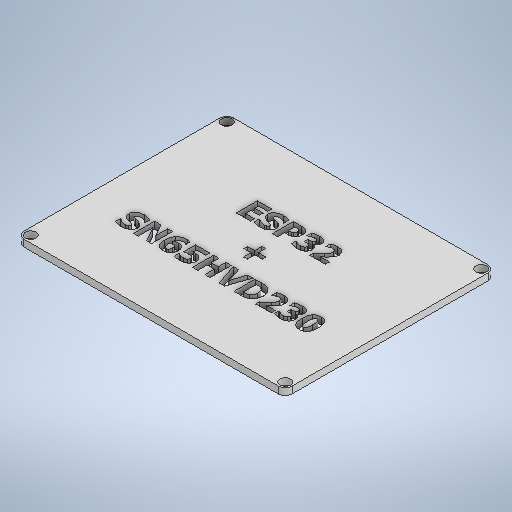
# Autodesk Inventor part: esp_can_case_lid
Saved by Autodesk Inventor 2025 (Build 290162000, 162)
## iProperties
Created: 2025-01-20
Part Number: esp_can_case_lid
Material: Generic
Document SubType Name: Modeling
Designer: danielrachi
Density: 1 g/cm^3
Appearance: Default
Author: danielrachi
Autodesk Inventor part; units mm, degrees
ref_plane "YZ Plane" through (0, 0, 0) normal (1, 0, 0) x (0, 1, 0)
ref_plane "XZ Plane" through (0, 0, 0) normal (0, 1, 0) x (-1, 0, 0)
ref_plane "XY Plane" through (0, 0, 0) normal (0, 0, 1) x (1, 0, 0)
sketch "Sketch1" plane through (0, 0, 0) normal (0, 1, 0) x (-1, 0, 0)
  line L0 (-39, 30.5) -> (39, 30.5)
  line L1 (39, 30.5) -> (39, -30.5)
  line L2 (39, -30.5) -> (-39, -30.5)
  line L3 (-39, -30.5) -> (-39, 30.5)
  line L4 (-39, 30.5) -> (39, -30.5) construction
  line L5 (39, 30.5) -> (-39, -30.5) construction
  point P0 (0, 0)
  dimension "d0" = 78
  dimension "d1" = 61
  constraints: 12 end point, 2 midpoint, 2 parallel, 1 horizontal, 1 perpendicular
  measures "d0" distance of L1.end L2.end
  measures "d1" distance of L0.end L1.end
extrude "Extrusion1" add sketch "Sketch1" along normal blind 2
sketch "Sketch2" plane through (0, 2, 0) normal (0, 1, 0) x (1, 0, 0)
  circle A0 centre (37, -28.5) radius 1.55
  line L0 (-39, -30.5) -> (39, -30.5) projected
  line L1 (39, -30.5) -> (39, 30.5) projected
  line L2 (-39, 30.5) -> (-39, -30.5) projected
  line L3 (-39, 0) -> (39, 0)
  line L4 (39, 30.5) -> (-39, 30.5) projected
  line L5 (0, 30.5) -> (0, -30.5)
  circle A1 centre (-37, -28.5) radius 1.55
  circle A2 centre (37, 28.5) radius 1.55
  circle A3 centre (-37, 28.5) radius 1.55
  line L6 (-39, 30.5) -> (39, 30.5) construction
  line L7 (39, 30.5) -> (39, -30.5) construction
  line L8 (39, -30.5) -> (-39, -30.5) construction
  line L9 (-39, -30.5) -> (-39, 30.5) construction
  line L10 (-12.7042, 6.9935) -> (-12.7042, 13.0935)
  line L11 (-12.7042, 13.0935) -> (-8.5815, 13.0935)
  line L12 (-8.5815, 13.0935) -> (-8.5815, 11.9318)
  line L13 (-8.5815, 11.9318) -> (-11.1817, 11.9318)
  line L14 (-11.1817, 11.9318) -> (-11.1817, 10.8591)
  line L15 (-11.1817, 10.8591) -> (-8.7842, 10.8591)
  line L16 (-8.7842, 10.8591) -> (-8.7842, 9.6975)
  line L17 (-8.7842, 9.6975) -> (-11.1817, 9.6975)
  line L18 (-11.1817, 9.6975) -> (-11.1817, 8.1552)
  line L19 (-11.1817, 8.1552) -> (-8.5815, 8.1552)
  line L20 (-8.5815, 8.1552) -> (-8.5815, 6.9935)
  line L21 (-8.5815, 6.9935) -> (-12.7042, 6.9935)
  spline S0 degree 2 poles (-5.66, 6.8847) (-6.362, 6.8847) (-7.4199, 7.1566) (-7.8746, 7.3543) knots 0 0 0 1 2 2 2
  line L22 (-7.8746, 7.3543) -> (-7.8746, 8.8077)
  line L23 (-7.8746, 8.8077) -> (-7.7362, 8.8077)
  spline S1 degree 2 poles (-7.7362, 8.8077) (-7.2765, 8.4172) (-6.1741, 7.997) (-5.6551, 7.997) knots 0 0 0 1 2 2 2
  spline S2 degree 2 poles (-5.6551, 7.997) (-5.5216, 7.997) (-5.0916, 8.0563) (-4.963, 8.1156) knots 0 0 0 1 2 2 2
  spline S3 degree 2 poles (-4.963, 8.1156) (-4.8049, 8.1848) (-4.5824, 8.4369) (-4.5824, 8.6396) knots 0 0 0 1 2 2 2
  spline S4 degree 2 poles (-4.5824, 8.6396) (-4.5824, 8.8719) (-4.9433, 9.1586) (-5.1904, 9.2229) knots 0 0 0 1 2 2 2
  spline S5 degree 2 poles (-5.1904, 9.2229) (-5.5019, 9.3069) (-6.2088, 9.4503) (-6.5202, 9.559) knots 0 0 0 1 2 2 2
  spline S6 degree 2 poles (-6.5202, 9.559) (-7.2271, 9.8062) (-7.84, 10.6515) (-7.84, 11.2843) knots 0 0 0 1 2 2 2
  spline S7 degree 2 poles (-7.84, 11.2843) (-7.84, 12.1394) (-6.3917, 13.2022) (-5.3041, 13.2022) knots 0 0 0 1 2 2 2
  spline S8 degree 2 poles (-5.3041, 13.2022) (-4.7604, 13.2022) (-3.6827, 12.9798) (-3.2576, 12.792) knots 0 0 0 1 2 2 2
  line L24 (-3.2576, 12.792) -> (-3.2576, 11.3979)
  line L25 (-3.2576, 11.3979) -> (-3.3911, 11.3979)
  spline S9 degree 2 poles (-3.3911, 11.3979) (-3.7322, 11.6896) (-4.7109, 12.09) (-5.225, 12.09) knots 0 0 0 1 2 2 2
  spline S10 degree 2 poles (-5.225, 12.09) (-5.4277, 12.09) (-5.7441, 12.0307) (-5.922, 11.9516) knots 0 0 0 1 2 2 2
  spline S11 degree 2 poles (-5.922, 11.9516) (-6.0654, 11.8873) (-6.273, 11.6303) (-6.273, 11.4721) knots 0 0 0 1 2 2 2
  spline S12 degree 2 poles (-6.273, 11.4721) (-6.273, 11.2348) (-5.9418, 10.9629) (-5.4673, 10.8542) knots 0 0 0 1 2 2 2
  spline S13 degree 2 poles (-5.4673, 10.8542) (-5.1608, 10.785) (-4.5923, 10.6515) (-4.266, 10.5378) knots 0 0 0 1 2 2 2
  spline S14 degree 2 poles (-4.266, 10.5378) (-3.6333, 10.3055) (-3.0154, 9.5343) (-3.0154, 8.9016) knots 0 0 0 1 2 2 2
  spline S15 degree 2 poles (-3.0154, 8.9016) (-3.0154, 7.992) (-4.444, 6.8847) (-5.66, 6.8847) knots 0 0 0 1 2 2 2
  spline S16 degree 2 poles (2.4618, 11.1706) (2.4618, 10.7454) (2.1899, 9.9743) (1.9378, 9.7172) knots 0 0 0 1 2 2 2
  spline S17 degree 2 poles (1.9378, 9.7172) (1.7845, 9.5541) (1.4088, 9.2872) (1.1864, 9.1932) knots 0 0 0 1 2 2 2
  spline S18 degree 2 poles (1.1864, 9.1932) (0.959, 9.0993) (0.4301, 8.9906) (0.1038, 8.9906) knots 0 0 0 1 2 2 2
  line L26 (0.1038, 8.9906) -> (-0.697, 8.9906)
  line L27 (-0.697, 8.9906) -> (-0.697, 6.9935)
  line L28 (-0.697, 6.9935) -> (-2.2294, 6.9935)
  line L29 (-2.2294, 6.9935) -> (-2.2294, 13.0935)
  line L30 (-2.2294, 13.0935) -> (0.1384, 13.0935)
  spline S19 degree 2 poles (0.1384, 13.0935) (0.6624, 13.0935) (1.4286, 12.9007) (1.74, 12.6931) knots 0 0 0 1 2 2 2
  spline S20 degree 2 poles (1.74, 12.6931) (2.0861, 12.4608) (2.4618, 11.6995) (2.4618, 11.1706) knots 0 0 0 1 2 2 2
  spline S21 degree 2 poles (0.8898, 11.131) (0.8898, 11.393) (0.6426, 11.7637) (0.4746, 11.833) knots 0 0 0 1 2 2 2
  spline S22 degree 2 poles (0.4746, 11.833) (0.2571, 11.9269) (-0.1384, 11.9565) (-0.4795, 11.9565) knots 0 0 0 1 2 2 2
  line L31 (-0.4795, 11.9565) -> (-0.697, 11.9565)
  line L32 (-0.697, 11.9565) -> (-0.697, 10.1275)
  line L33 (-0.697, 10.1275) -> (-0.5882, 10.1275)
  spline S23 degree 2 poles (-0.5882, 10.1275) (-0.3757, 10.1275) (0.0099, 10.1374) (0.1532, 10.1621) knots 0 0 0 1 2 2 2
  spline S24 degree 2 poles (0.1532, 10.1621) (0.2768, 10.1819) (0.5487, 10.3005) (0.6229, 10.3747) knots 0 0 0 1 2 2 2
  spline S25 degree 2 poles (0.6229, 10.3747) (0.781, 10.523) (0.8898, 10.8542) (0.8898, 11.131) knots 0 0 0 1 2 2 2
  spline S26 degree 2 poles (7.5978, 8.8423) (7.5978, 8.3924) (7.2666, 7.6559) (6.9453, 7.3988) knots 0 0 0 1 2 2 2
  spline S27 degree 2 poles (6.9453, 7.3988) (6.624, 7.1418) (5.749, 6.865) (5.1212, 6.865) knots 0 0 0 1 2 2 2
  spline S28 degree 2 poles (5.1212, 6.865) (4.4094, 6.865) (3.3911, 7.1022) (3.0698, 7.2505) knots 0 0 0 1 2 2 2
  line L34 (3.0698, 7.2505) -> (3.0698, 8.5753)
  line L35 (3.0698, 8.5753) -> (3.2181, 8.5753)
  spline S29 degree 2 poles (3.2181, 8.5753) (3.5542, 8.3628) (4.4588, 8.0464) (4.8345, 8.0464) knots 0 0 0 1 2 2 2
  spline S30 degree 2 poles (4.8345, 8.0464) (5.057, 8.0464) (5.576, 8.1255) (5.754, 8.254) knots 0 0 0 1 2 2 2
  spline S31 degree 2 poles (5.754, 8.254) (5.8924, 8.3578) (6.0605, 8.6594) (6.0605, 8.9313) knots 0 0 0 1 2 2 2
  spline S32 degree 2 poles (6.0605, 8.9313) (6.0605, 9.2031) (5.8232, 9.4948) (5.6254, 9.564) knots 0 0 0 1 2 2 2
  spline S33 degree 2 poles (5.6254, 9.564) (5.4277, 9.6332) (4.879, 9.648) (4.6665, 9.648) knots 0 0 0 1 2 2 2
  line L36 (4.6665, 9.648) -> (4.4045, 9.648)
  line L37 (4.4045, 9.648) -> (4.4045, 10.7207)
  line L38 (4.4045, 10.7207) -> (4.6467, 10.7207)
  spline S34 degree 2 poles (4.6467, 10.7207) (4.9235, 10.7207) (5.3931, 10.7702) (5.5562, 10.8443) knots 0 0 0 1 2 2 2
  spline S35 degree 2 poles (5.5562, 10.8443) (5.7194, 10.9234) (5.9023, 11.2002) (5.9023, 11.4375) knots 0 0 0 1 2 2 2
  spline S36 degree 2 poles (5.9023, 11.4375) (5.9023, 11.6253) (5.7293, 11.8577) (5.6057, 11.9219) knots 0 0 0 1 2 2 2
  spline S37 degree 2 poles (5.6057, 11.9219) (5.4574, 11.9961) (5.0619, 12.0455) (4.9235, 12.0455) knots 0 0 0 1 2 2 2
  spline S38 degree 2 poles (4.9235, 12.0455) (4.7011, 12.0455) (4.2314, 11.9417) (4.0139, 11.8577) knots 0 0 0 1 2 2 2
  spline S39 degree 2 poles (4.0139, 11.8577) (3.8409, 11.7934) (3.4652, 11.5858) (3.3763, 11.5314) knots 0 0 0 1 2 2 2
  line L39 (3.3763, 11.5314) -> (3.2477, 11.5314)
  line L40 (3.2477, 11.5314) -> (3.2477, 12.8364)
  spline S40 degree 2 poles (3.2477, 12.8364) (3.5641, 12.9699) (4.6318, 13.222) (5.1904, 13.222) knots 0 0 0 1 2 2 2
  spline S41 degree 2 poles (5.1904, 13.222) (5.7342, 13.222) (6.535, 13.0342) (6.8168, 12.8513) knots 0 0 0 1 2 2 2
  spline S42 degree 2 poles (6.8168, 12.8513) (7.1282, 12.6585) (7.4396, 12.0653) (7.4396, 11.6945) knots 0 0 0 1 2 2 2
  spline S43 degree 2 poles (7.4396, 11.6945) (7.4396, 11.1706) (6.8365, 10.3895) (6.3422, 10.2758) knots 0 0 0 1 2 2 2
  line L41 (6.3422, 10.2758) -> (6.3422, 10.2165)
  spline S44 degree 2 poles (6.3422, 10.2165) (6.5597, 10.1868) (6.975, 10.0287) (7.1727, 9.8507) knots 0 0 0 1 2 2 2
  spline S45 degree 2 poles (7.1727, 9.8507) (7.3556, 9.6925) (7.5978, 9.1883) (7.5978, 8.8423) knots 0 0 0 1 2 2 2
  line L42 (13.0947, 6.9935) -> (8.6112, 6.9935)
  line L43 (8.6112, 6.9935) -> (8.6112, 7.9871)
  spline S46 degree 2 poles (8.6112, 7.9871) (9.1797, 8.4419) (10.0892, 9.2427) (10.4303, 9.6035) knots 0 0 0 1 2 2 2
  spline S47 degree 2 poles (10.4303, 9.6035) (10.8801, 10.0731) (11.2806, 10.7899) (11.2806, 11.1656) knots 0 0 0 1 2 2 2
  spline S48 degree 2 poles (11.2806, 11.1656) (11.2806, 11.5907) (10.7714, 12.0455) (10.3166, 12.0455) knots 0 0 0 1 2 2 2
  spline S49 degree 2 poles (10.3166, 12.0455) (10.0843, 12.0455) (9.669, 11.9318) (9.4565, 11.8428) knots 0 0 0 1 2 2 2
  spline S50 degree 2 poles (9.4565, 11.8428) (9.2489, 11.7489) (8.9523, 11.5512) (8.8781, 11.5018) knots 0 0 0 1 2 2 2
  line L44 (8.8781, 11.5018) -> (8.7595, 11.5018)
  line L45 (8.7595, 11.5018) -> (8.7595, 12.8315)
  spline S51 degree 2 poles (8.7595, 12.8315) (9.0165, 12.9551) (10.1139, 13.2121) (10.6231, 13.2121) knots 0 0 0 1 2 2 2
  spline S52 degree 2 poles (10.6231, 13.2121) (11.7106, 13.2121) (12.8278, 12.2432) (12.8278, 11.3683) knots 0 0 0 1 2 2 2
  spline S53 degree 2 poles (12.8278, 11.3683) (12.8278, 10.8295) (12.3186, 9.7914) (11.7304, 9.1982) knots 0 0 0 1 2 2 2
  spline S54 degree 2 poles (11.7304, 9.1982) (11.3596, 8.8324) (10.6626, 8.2639) (10.5094, 8.1453) knots 0 0 0 1 2 2 2
  line L46 (10.5094, 8.1453) -> (13.0947, 8.1453)
  line L47 (13.0947, 8.1453) -> (13.0947, 6.9935)
  line L48 (2.6372, -0.8898) -> (0.5413, -0.8898)
  line L49 (0.5413, -0.8898) -> (0.5413, -2.9709)
  line L50 (0.5413, -2.9709) -> (-0.5413, -2.9709)
  line L51 (-0.5413, -2.9709) -> (-0.5413, -0.8898)
  line L52 (-0.5413, -0.8898) -> (-2.6372, -0.8898)
  line L53 (-2.6372, -0.8898) -> (-2.6372, 0.1681)
  line L54 (-2.6372, 0.1681) -> (-0.5413, 0.1681)
  line L55 (-0.5413, 0.1681) -> (-0.5413, 2.2492)
  line L56 (-0.5413, 2.2492) -> (0.5413, 2.2492)
  line L57 (0.5413, 2.2492) -> (0.5413, 0.1681)
  line L58 (0.5413, 0.1681) -> (2.6372, 0.1681)
  line L59 (2.6372, 0.1681) -> (2.6372, -0.8898)
  spline S55 degree 2 poles (-25.9448, -13.2022) (-26.6467, -13.2022) (-27.7046, -12.9304) (-28.1594, -12.7326) knots 0 0 0 1 2 2 2
  line L60 (-28.1594, -12.7326) -> (-28.1594, -11.2793)
  line L61 (-28.1594, -11.2793) -> (-28.0209, -11.2793)
  spline S56 degree 2 poles (-28.0209, -11.2793) (-27.5612, -11.6698) (-26.4589, -12.09) (-25.9398, -12.09) knots 0 0 0 1 2 2 2
  spline S57 degree 2 poles (-25.9398, -12.09) (-25.8064, -12.09) (-25.3763, -12.0307) (-25.2478, -11.9714) knots 0 0 0 1 2 2 2
  spline S58 degree 2 poles (-25.2478, -11.9714) (-25.0896, -11.9022) (-24.8671, -11.6501) (-24.8671, -11.4474) knots 0 0 0 1 2 2 2
  spline S59 degree 2 poles (-24.8671, -11.4474) (-24.8671, -11.215) (-25.228, -10.9283) (-25.4752, -10.8641) knots 0 0 0 1 2 2 2
  spline S60 degree 2 poles (-25.4752, -10.8641) (-25.7866, -10.78) (-26.4935, -10.6367) (-26.8049, -10.5279) knots 0 0 0 1 2 2 2
  spline S61 degree 2 poles (-26.8049, -10.5279) (-27.5118, -10.2808) (-28.1248, -9.4355) (-28.1248, -8.8027) knots 0 0 0 1 2 2 2
  spline S62 degree 2 poles (-28.1248, -8.8027) (-28.1248, -7.9475) (-26.6764, -6.8847) (-25.5889, -6.8847) knots 0 0 0 1 2 2 2
  spline S63 degree 2 poles (-25.5889, -6.8847) (-25.0451, -6.8847) (-23.9675, -7.1072) (-23.5423, -7.295) knots 0 0 0 1 2 2 2
  line L62 (-23.5423, -7.295) -> (-23.5423, -8.689)
  line L63 (-23.5423, -8.689) -> (-23.6758, -8.689)
  spline S64 degree 2 poles (-23.6758, -8.689) (-24.0169, -8.3974) (-24.9957, -7.997) (-25.5098, -7.997) knots 0 0 0 1 2 2 2
  spline S65 degree 2 poles (-25.5098, -7.997) (-25.7124, -7.997) (-26.0288, -8.0563) (-26.2068, -8.1354) knots 0 0 0 1 2 2 2
  spline S66 degree 2 poles (-26.2068, -8.1354) (-26.3501, -8.1996) (-26.5577, -8.4567) (-26.5577, -8.6149) knots 0 0 0 1 2 2 2
  spline S67 degree 2 poles (-26.5577, -8.6149) (-26.5577, -8.8522) (-26.2265, -9.124) (-25.752, -9.2328) knots 0 0 0 1 2 2 2
  spline S68 degree 2 poles (-25.752, -9.2328) (-25.4455, -9.302) (-24.877, -9.4355) (-24.5508, -9.5492) knots 0 0 0 1 2 2 2
  spline S69 degree 2 poles (-24.5508, -9.5492) (-23.918, -9.7815) (-23.3001, -10.5526) (-23.3001, -11.1854) knots 0 0 0 1 2 2 2
  spline S70 degree 2 poles (-23.3001, -11.1854) (-23.3001, -12.0949) (-24.7287, -13.2022) (-25.9448, -13.2022) knots 0 0 0 1 2 2 2
  line L64 (-17.2891, -13.0935) -> (-18.7622, -13.0935)
  line L65 (-18.7622, -13.0935) -> (-21.1152, -8.8423)
  line L66 (-21.1152, -8.8423) -> (-21.1152, -13.0935)
  line L67 (-21.1152, -13.0935) -> (-22.5141, -13.0935)
  line L68 (-22.5141, -13.0935) -> (-22.5141, -6.9935)
  line L69 (-22.5141, -6.9935) -> (-20.6357, -6.9935)
  line L70 (-20.6357, -6.9935) -> (-18.688, -10.4884)
  line L71 (-18.688, -10.4884) -> (-18.688, -6.9935)
  line L72 (-18.688, -6.9935) -> (-17.2891, -6.9935)
  line L73 (-17.2891, -6.9935) -> (-17.2891, -13.0935)
  spline S71 degree 2 poles (-11.6142, -11.0173) (-11.6142, -11.9813) (-12.8352, -13.222) (-13.903, -13.222) knots 0 0 0 1 2 2 2
  spline S72 degree 2 poles (-13.903, -13.222) (-14.4368, -13.222) (-15.2722, -12.9155) (-15.5639, -12.614) knots 0 0 0 1 2 2 2
  spline S73 degree 2 poles (-15.5639, -12.614) (-15.9099, -12.263) (-16.2807, -11.1508) (-16.2807, -10.3747) knots 0 0 0 1 2 2 2
  spline S74 degree 2 poles (-16.2807, -10.3747) (-16.2807, -9.5739) (-15.9346, -8.3282) (-15.5441, -7.8487) knots 0 0 0 1 2 2 2
  spline S75 degree 2 poles (-15.5441, -7.8487) (-15.1734, -7.3939) (-13.9672, -6.8798) (-13.1417, -6.8798) knots 0 0 0 1 2 2 2
  spline S76 degree 2 poles (-13.1417, -6.8798) (-12.8402, -6.8798) (-12.2371, -6.9589) (-12.1283, -6.9836) knots 0 0 0 1 2 2 2
  line L74 (-12.1283, -6.9836) -> (-12.1283, -8.1799)
  line L75 (-12.1283, -8.1799) -> (-12.2371, -8.1799)
  spline S77 degree 2 poles (-12.2371, -8.1799) (-12.3458, -8.1255) (-12.8402, -7.992) (-13.1565, -7.992) knots 0 0 0 1 2 2 2
  spline S78 degree 2 poles (-13.1565, -7.992) (-13.8733, -7.992) (-14.6543, -8.7484) (-14.7483, -9.4503) knots 0 0 0 1 2 2 2
  spline S79 degree 2 poles (-14.7483, -9.4503) (-14.4467, -9.2575) (-13.8288, -9.0301) (-13.4383, -9.0301) knots 0 0 0 1 2 2 2
  spline S80 degree 2 poles (-13.4383, -9.0301) (-13.1071, -9.0301) (-12.5287, -9.2081) (-12.3063, -9.3761) knots 0 0 0 1 2 2 2
  spline S81 degree 2 poles (-12.3063, -9.3761) (-11.9899, -9.6184) (-11.6142, -10.4043) (-11.6142, -11.0173) knots 0 0 0 1 2 2 2
  spline S82 degree 2 poles (-13.3987, -11.9368) (-13.2801, -11.7885) (-13.1516, -11.4424) (-13.1516, -11.0915) knots 0 0 0 1 2 2 2
  spline S83 degree 2 poles (-13.1516, -11.0915) (-13.1516, -10.7949) (-13.2999, -10.4093) (-13.4333, -10.2956) knots 0 0 0 1 2 2 2
  spline S84 degree 2 poles (-13.4333, -10.2956) (-13.5718, -10.177) (-13.9128, -10.0929) (-14.1056, -10.0929) knots 0 0 0 1 2 2 2
  spline S85 degree 2 poles (-14.1056, -10.0929) (-14.2688, -10.0929) (-14.6049, -10.177) (-14.7532, -10.2363) knots 0 0 0 1 2 2 2
  spline S86 degree 2 poles (-14.7532, -10.2363) (-14.7532, -10.2758) (-14.7631, -10.4637) (-14.7631, -10.607) knots 0 0 0 1 2 2 2
  spline S87 degree 2 poles (-14.7631, -10.607) (-14.7631, -11.136) (-14.5802, -11.7736) (-14.4368, -11.9368) knots 0 0 0 1 2 2 2
  spline S88 degree 2 poles (-14.4368, -11.9368) (-14.333, -12.0702) (-14.0562, -12.1839) (-13.9079, -12.1839) knots 0 0 0 1 2 2 2
  spline S89 degree 2 poles (-13.9079, -12.1839) (-13.7843, -12.1839) (-13.4976, -12.0603) (-13.3987, -11.9368) knots 0 0 0 1 2 2 2
  spline S90 degree 2 poles (-6.3744, -11.0272) (-6.3744, -11.5067) (-6.7006, -12.3174) (-7.0219, -12.609) knots 0 0 0 1 2 2 2
  spline S91 degree 2 poles (-7.0219, -12.609) (-7.3432, -12.9007) (-8.2231, -13.222) (-8.8658, -13.222) knots 0 0 0 1 2 2 2
  spline S92 degree 2 poles (-8.8658, -13.222) (-9.5479, -13.2171) (-10.5267, -12.9946) (-10.848, -12.8513) knots 0 0 0 1 2 2 2
  line L76 (-10.848, -12.8513) -> (-10.848, -11.5215)
  line L77 (-10.848, -11.5215) -> (-10.7096, -11.5215)
  spline S93 degree 2 poles (-10.7096, -11.5215) (-10.591, -11.5858) (-10.3043, -11.7539) (-10.0719, -11.8428) knots 0 0 0 1 2 2 2
  spline S94 degree 2 poles (-10.0719, -11.8428) (-9.8544, -11.9269) (-9.4046, -12.0406) (-9.1327, -12.0406) knots 0 0 0 1 2 2 2
  spline S95 degree 2 poles (-9.1327, -12.0406) (-8.8954, -12.0406) (-8.3418, -11.9219) (-8.1737, -11.7637) knots 0 0 0 1 2 2 2
  spline S96 degree 2 poles (-8.1737, -11.7637) (-8.0501, -11.6402) (-7.9117, -11.3386) (-7.9117, -11.0865) knots 0 0 0 1 2 2 2
  spline S97 degree 2 poles (-7.9117, -11.0865) (-7.9117, -10.869) (-8.0897, -10.5625) (-8.233, -10.4686) knots 0 0 0 1 2 2 2
  spline S98 degree 2 poles (-8.233, -10.4686) (-8.4406, -10.3302) (-9.0338, -10.2511) (-9.2464, -10.2511) knots 0 0 0 1 2 2 2
  spline S99 degree 2 poles (-9.2464, -10.2511) (-9.5825, -10.2511) (-10.2202, -10.3599) (-10.4526, -10.4192) knots 0 0 0 1 2 2 2
  line L78 (-10.4526, -10.4192) -> (-10.586, -10.4192)
  line L79 (-10.586, -10.4192) -> (-10.586, -6.9935)
  line L80 (-10.586, -6.9935) -> (-6.5424, -6.9935)
  line L81 (-6.5424, -6.9935) -> (-6.5424, -8.1453)
  line L82 (-6.5424, -8.1453) -> (-9.1376, -8.1453)
  line L83 (-9.1376, -8.1453) -> (-9.1376, -9.1586)
  spline S100 degree 2 poles (-9.1376, -9.1586) (-9.0141, -9.1488) (-8.673, -9.1389) (-8.5791, -9.1389) knots 0 0 0 1 2 2 2
  spline S101 degree 2 poles (-8.5791, -9.1389) (-8.1391, -9.1389) (-7.3976, -9.3168) (-7.106, -9.4997) knots 0 0 0 1 2 2 2
  spline S102 degree 2 poles (-7.106, -9.4997) (-6.7599, -9.7271) (-6.3744, -10.4834) (-6.3744, -11.0272) knots 0 0 0 1 2 2 2
  line L84 (-0.215, -13.0935) -> (-1.7474, -13.0935)
  line L85 (-1.7474, -13.0935) -> (-1.7474, -10.3895)
  line L86 (-1.7474, -10.3895) -> (-3.8286, -10.3895)
  line L87 (-3.8286, -10.3895) -> (-3.8286, -13.0935)
  line L88 (-3.8286, -13.0935) -> (-5.361, -13.0935)
  line L89 (-5.361, -13.0935) -> (-5.361, -6.9935)
  line L90 (-5.361, -6.9935) -> (-3.8286, -6.9935)
  line L91 (-3.8286, -6.9935) -> (-3.8286, -9.2278)
  line L92 (-3.8286, -9.2278) -> (-1.7474, -9.2278)
  line L93 (-1.7474, -9.2278) -> (-1.7474, -6.9935)
  line L94 (-1.7474, -6.9935) -> (-0.215, -6.9935)
  line L95 (-0.215, -6.9935) -> (-0.215, -13.0935)
  line L96 (6.142, -6.9935) -> (4.0461, -13.0935)
  line L97 (4.0461, -13.0935) -> (2.4494, -13.0935)
  line L98 (2.4494, -13.0935) -> (0.3534, -6.9935)
  line L99 (0.3534, -6.9935) -> (1.9402, -6.9935)
  line L100 (1.9402, -6.9935) -> (3.27, -11.131)
  line L101 (3.27, -11.131) -> (4.5948, -6.9935)
  line L102 (4.5948, -6.9935) -> (6.142, -6.9935)
  spline S103 degree 2 poles (12.153, -10.0484) (12.153, -10.9036) (11.4066, -12.2482) (10.8381, -12.609) knots 0 0 0 1 2 2 2
  spline S104 degree 2 poles (10.8381, -12.609) (10.3636, -12.9155) (9.2464, -13.0935) (8.6186, -13.0935) knots 0 0 0 1 2 2 2
  line L103 (8.6186, -13.0935) -> (6.7105, -13.0935)
  line L104 (6.7105, -13.0935) -> (6.7105, -6.9935)
  line L105 (6.7105, -6.9935) -> (8.5988, -6.9935)
  spline S105 degree 2 poles (8.5988, -6.9935) (9.2415, -6.9935) (10.3636, -7.1566) (10.8579, -7.473) knots 0 0 0 1 2 2 2
  spline S106 degree 2 poles (10.8579, -7.473) (11.456, -7.8586) (12.153, -9.1636) (12.153, -10.0484) knots 0 0 0 1 2 2 2
  spline S107 degree 2 poles (10.5811, -10.0385) (10.5811, -9.4355) (10.1658, -8.5753) (9.7407, -8.3331) knots 0 0 0 1 2 2 2
  spline S108 degree 2 poles (9.7407, -8.3331) (9.4293, -8.165) (8.7471, -8.1304) (8.2726, -8.1304) knots 0 0 0 1 2 2 2
  line L106 (8.2726, -8.1304) -> (8.2429, -8.1304)
  line L107 (8.2429, -8.1304) -> (8.2429, -11.9516)
  line L108 (8.2429, -11.9516) -> (8.2726, -11.9516)
  spline S109 degree 2 poles (8.2726, -11.9516) (8.7867, -11.9516) (9.4936, -11.917) (9.8149, -11.7143) knots 0 0 0 1 2 2 2
  spline S110 degree 2 poles (9.8149, -11.7143) (10.1906, -11.477) (10.5811, -10.6416) (10.5811, -10.0385) knots 0 0 0 1 2 2 2
  line L109 (17.5313, -13.0935) -> (13.0478, -13.0935)
  line L110 (13.0478, -13.0935) -> (13.0478, -12.0999)
  spline S111 degree 2 poles (13.0478, -12.0999) (13.6162, -11.6451) (14.5258, -10.8443) (14.8669, -10.4834) knots 0 0 0 1 2 2 2
  spline S112 degree 2 poles (14.8669, -10.4834) (15.3167, -10.0138) (15.7171, -9.2971) (15.7171, -8.9214) knots 0 0 0 1 2 2 2
  spline S113 degree 2 poles (15.7171, -8.9214) (15.7171, -8.4962) (15.208, -8.0415) (14.7532, -8.0415) knots 0 0 0 1 2 2 2
  spline S114 degree 2 poles (14.7532, -8.0415) (14.5209, -8.0415) (14.1056, -8.1552) (13.8931, -8.2441) knots 0 0 0 1 2 2 2
  spline S115 degree 2 poles (13.8931, -8.2441) (13.6855, -8.3381) (13.3889, -8.5358) (13.3147, -8.5852) knots 0 0 0 1 2 2 2
  line L111 (13.3147, -8.5852) -> (13.1961, -8.5852)
  line L112 (13.1961, -8.5852) -> (13.1961, -7.2555)
  spline S116 degree 2 poles (13.1961, -7.2555) (13.4531, -7.1319) (14.5505, -6.8749) (15.0597, -6.8749) knots 0 0 0 1 2 2 2
  spline S117 degree 2 poles (15.0597, -6.8749) (16.1472, -6.8749) (17.2644, -7.8437) (17.2644, -8.7187) knots 0 0 0 1 2 2 2
  spline S118 degree 2 poles (17.2644, -8.7187) (17.2644, -9.2575) (16.7552, -10.2956) (16.167, -10.8888) knots 0 0 0 1 2 2 2
  spline S119 degree 2 poles (16.167, -10.8888) (15.7962, -11.2546) (15.0992, -11.8231) (14.946, -11.9417) knots 0 0 0 1 2 2 2
  line L113 (14.946, -11.9417) -> (17.5313, -11.9417)
  line L114 (17.5313, -11.9417) -> (17.5313, -13.0935)
  spline S120 degree 2 poles (22.7218, -11.2447) (22.7218, -11.6945) (22.3906, -12.4311) (22.0692, -12.6881) knots 0 0 0 1 2 2 2
  spline S121 degree 2 poles (22.0692, -12.6881) (21.7479, -12.9452) (20.873, -13.222) (20.2452, -13.222) knots 0 0 0 1 2 2 2
  spline S122 degree 2 poles (20.2452, -13.222) (19.5333, -13.222) (18.515, -12.9847) (18.1937, -12.8364) knots 0 0 0 1 2 2 2
  line L115 (18.1937, -12.8364) -> (18.1937, -11.5116)
  line L116 (18.1937, -11.5116) -> (18.342, -11.5116)
  spline S123 degree 2 poles (18.342, -11.5116) (18.6782, -11.7242) (19.5828, -12.0406) (19.9585, -12.0406) knots 0 0 0 1 2 2 2
  spline S124 degree 2 poles (19.9585, -12.0406) (20.1809, -12.0406) (20.7, -11.9615) (20.8779, -11.833) knots 0 0 0 1 2 2 2
  spline S125 degree 2 poles (20.8779, -11.833) (21.0163, -11.7291) (21.1844, -11.4276) (21.1844, -11.1557) knots 0 0 0 1 2 2 2
  spline S126 degree 2 poles (21.1844, -11.1557) (21.1844, -10.8838) (20.9471, -10.5922) (20.7494, -10.523) knots 0 0 0 1 2 2 2
  spline S127 degree 2 poles (20.7494, -10.523) (20.5517, -10.4538) (20.003, -10.439) (19.7904, -10.439) knots 0 0 0 1 2 2 2
  line L117 (19.7904, -10.439) -> (19.5284, -10.439)
  line L118 (19.5284, -10.439) -> (19.5284, -9.3663)
  line L119 (19.5284, -9.3663) -> (19.7706, -9.3663)
  spline S128 degree 2 poles (19.7706, -9.3663) (20.0474, -9.3663) (20.5171, -9.3168) (20.6802, -9.2427) knots 0 0 0 1 2 2 2
  spline S129 degree 2 poles (20.6802, -9.2427) (20.8433, -9.1636) (21.0262, -8.8868) (21.0262, -8.6495) knots 0 0 0 1 2 2 2
  spline S130 degree 2 poles (21.0262, -8.6495) (21.0262, -8.4616) (20.8532, -8.2293) (20.7296, -8.165) knots 0 0 0 1 2 2 2
  spline S131 degree 2 poles (20.7296, -8.165) (20.5813, -8.0909) (20.1859, -8.0415) (20.0474, -8.0415) knots 0 0 0 1 2 2 2
  spline S132 degree 2 poles (20.0474, -8.0415) (19.825, -8.0415) (19.3554, -8.1453) (19.1379, -8.2293) knots 0 0 0 1 2 2 2
  spline S133 degree 2 poles (19.1379, -8.2293) (18.9649, -8.2936) (18.5892, -8.5012) (18.5002, -8.5556) knots 0 0 0 1 2 2 2
  line L120 (18.5002, -8.5556) -> (18.3717, -8.5556)
  line L121 (18.3717, -8.5556) -> (18.3717, -7.2505)
  spline S134 degree 2 poles (18.3717, -7.2505) (18.688, -7.1171) (19.7558, -6.865) (20.3144, -6.865) knots 0 0 0 1 2 2 2
  spline S135 degree 2 poles (20.3144, -6.865) (20.8581, -6.865) (21.659, -7.0528) (21.9407, -7.2357) knots 0 0 0 1 2 2 2
  spline S136 degree 2 poles (21.9407, -7.2357) (22.2521, -7.4285) (22.5636, -8.0217) (22.5636, -8.3924) knots 0 0 0 1 2 2 2
  spline S137 degree 2 poles (22.5636, -8.3924) (22.5636, -8.9164) (21.9605, -9.6975) (21.4662, -9.8112) knots 0 0 0 1 2 2 2
  line L122 (21.4662, -9.8112) -> (21.4662, -9.8705)
  spline S138 degree 2 poles (21.4662, -9.8705) (21.6837, -9.9001) (22.0989, -10.0583) (22.2966, -10.2363) knots 0 0 0 1 2 2 2
  spline S139 degree 2 poles (22.2966, -10.2363) (22.4795, -10.3945) (22.7218, -10.8987) (22.7218, -11.2447) knots 0 0 0 1 2 2 2
  spline S140 degree 2 poles (28.1396, -10.0435) (28.1396, -10.8344) (27.8875, -12.0208) (27.6057, -12.4212) knots 0 0 0 1 2 2 2
  spline S141 degree 2 poles (27.6057, -12.4212) (27.3289, -12.8167) (26.4342, -13.222) (25.7915, -13.222) knots 0 0 0 1 2 2 2
  spline S142 degree 2 poles (25.7915, -13.222) (25.144, -13.222) (24.2542, -12.8167) (23.9724, -12.4113) knots 0 0 0 1 2 2 2
  spline S143 degree 2 poles (23.9724, -12.4113) (23.6906, -12.0109) (23.4385, -10.8344) (23.4385, -10.0435) knots 0 0 0 1 2 2 2
  spline S144 degree 2 poles (23.4385, -10.0435) (23.4385, -9.2328) (23.6906, -8.086) (23.9774, -7.6707) knots 0 0 0 1 2 2 2
  spline S145 degree 2 poles (23.9774, -7.6707) (24.2641, -7.2654) (25.1687, -6.8699) (25.7915, -6.8699) knots 0 0 0 1 2 2 2
  spline S146 degree 2 poles (25.7915, -6.8699) (26.449, -6.8699) (27.3289, -7.2851) (27.6107, -7.6954) knots 0 0 0 1 2 2 2
  spline S147 degree 2 poles (27.6107, -7.6954) (27.8875, -8.0958) (28.1396, -9.2773) (28.1396, -10.0435) knots 0 0 0 1 2 2 2
  spline S148 degree 2 poles (26.6022, -10.0435) (26.6022, -8.9115) (26.2315, -7.997) (25.7915, -7.997) knots 0 0 0 1 2 2 2
  spline S149 degree 2 poles (25.7915, -7.997) (25.3516, -7.997) (24.9759, -8.9115) (24.9759, -10.0484) knots 0 0 0 1 2 2 2
  spline S150 degree 2 poles (24.9759, -10.0484) (24.9759, -11.1656) (25.3516, -12.0949) (25.7915, -12.0949) knots 0 0 0 1 2 2 2
  spline S151 degree 2 poles (25.7915, -12.0949) (26.2265, -12.0949) (26.6022, -11.1656) (26.6022, -10.0435) knots 0 0 0 1 2 2 2
  point P0 (0, 0)
  dimension "d4" = 3.1
  dimension "d5" = 2
  dimension "d6" = 2
  constraints: 4 centre point, 4 collinear, 4 end point, 4 midpoint, 3 symmetric about line, 5 other
  measures "d4" diameter of A0
  measures "d5" distance from line of A0.centre L0
  measures "d6" distance from line of A0.centre L1
extrude "Extrusion2" cut sketch "Sketch2" against normal up to next contours A0 | L50 L51 L52 L53 L3 L5 | L5 L3 L59 L48 L49 L50 | L53 L54 L55 L56 L5 L3 | L5 L56 L57 L58 L59 L3 | L30 S19 S20 S16 S17 S18 L26 L5 S23 S24 S25 S21 S22 | L5 S22 L31 L32 L33 S23 L26 L27 L28 L29 L30 | A1 | A2 | A3 | L10 L11 L12 L13 L14 L15 L16 L17 L18 L19 L20 L21 | S0 L22 L23 S1 S2 S3 S4 S5 S6 S7 S8 L24 L25 S9 S10 S11 S12 S13 S14 S15 | S26 S27 S28 L34 L35 S29 S30 S31 S32 S33 L36 L37 L38 S34 S35 S36 S37 S38 S39 L39 L40 S40 S41 S42 S43 L41 S44 S45 | L42 L43 S46 S47 S48 S49 S50 L44 L45 S51 S52 S53 S54 L46 L47 | S55 L60 L61 S56 S57 S58 S59 S60 S61 S62 S63 L62 L63 S64 S65 S66 S67 S68 S69 S70 | L64 L65 L66 L67 L68 L69 L70 L71 L72 L73 | S71 S72 S73 S74 S75 S76 L74 L75 S77 S78 S79 S80 S81 | S90 S91 S92 L76 L77 S93 S94 S95 S96 S97 S98 S99 L78 L79 L80 L81 L82 L83 S100 S101 S102 | L84 L85 L86 L87 L88 L89 L90 L91 L92 L93 L94 L95 | L96 L97 L98 L99 L100 L101 L102 | S103 S104 L103 L104 L105 S105 S106 | L109 L110 S111 S112 S113 S114 S115 L111 L112 S116 S117 S118 S119 L113 L114 | S120 S121 S122 L115 L116 S123 S124 S125 S126 S127 L117 L118 L119 S128 S129 S130 S131 S132 S133 L120 L121 S134 S135 S136 S137 L122 S138 S139 | S140 S141 S142 S143 S144 S145 S146 S147
fillet "Fillet1" radius 2 4 edges at (-39, 1, 30.5) (39, 1, 30.5) (39, 1, -30.5) (-39, 1, -30.5)
body "Solid1"
